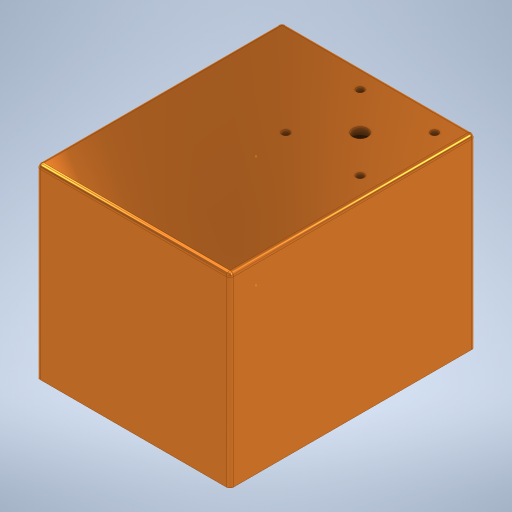
# Autodesk Inventor part: case
Saved by Autodesk Inventor 2023 (Build 270158000, 158)
## iProperties
Created: 2022-11-26
Part Number: case
Material: Gold
Document SubType Name: Modeling
Designer: abdul
Density: 19.3 g/cm^3
Appearance: Metal 1600F Hot
Author: abdul
Autodesk Inventor part; units mm, degrees
ref_plane "YZ Plane" through (0, 0, 0) normal (1, 0, 0) x (0, 1, 0)
ref_plane "XZ Plane" through (0, 0, 0) normal (0, 1, 0) x (-1, 0, 0)
ref_plane "XY Plane" through (0, 0, 0) normal (0, 0, 1) x (1, 0, 0)
sketch "Sketch1" plane through (0, 0, 0) normal (0, 1, 0) x (-1, 0, 0)
  line L0 (130, 165) -> (-130, 165)
  line L1 (-130, 165) -> (-130, -165)
  line L2 (-130, -165) -> (130, -165)
  line L3 (130, -165) -> (130, 165)
  point P0 (0, 0)
  point P1 (0, -165)
  point P2 (-130, 0)
  dimension "d0" = 260
  dimension "d1" = 330
  constraints: 8 end point, 2 midpoint, 2 parallel, 1 horizontal, 1 horizontal alignment, 1 perpendicular, 1 vertical alignment
  measures "d0" distance of L2.end L1.end
  measures "d1" distance of L1.end L0.end
extrude "Extrusion1" add sketch "Sketch1" along normal blind 250
sketch "Sketch2" plane through (0, 0, 0) normal (0, -1, 0) x (1, 0, 0)
  line L0 (-120, 155) -> (120, 155)
  line L1 (120, 155) -> (120, -155)
  line L2 (120, -155) -> (-120, -155)
  line L3 (-120, -155) -> (-120, 155)
  line L4 (-130, 165) -> (130, 165) projected
  line L5 (130, 165) -> (130, -165) projected
  point P0 (0, 0)
  point P1 (0, 155)
  point P2 (-120, 0)
  dimension "d4" = 10
  dimension "d5" = 10
  constraints: 8 end point, 2 midpoint, 2 parallel, 1 horizontal, 1 horizontal alignment, 1 perpendicular, 1 vertical alignment
  measures "d4" distance between parallel lines of L4 L0
  measures "d5" distance between parallel lines of L5 L1
extrude "Extrusion2" cut sketch "Sketch2" against normal blind 240
fillet "Fillet1" radius 5 8 edges at (0, 250, 165) (-130, 250, 0) (130, 250, 0) (0, 250, -165) (130, 125, -165) (130, 125, 165) (-130, 125, 165) (-130, 125, -165)
sketch "Sketch3" plane through (0, 250, 0) normal (0, 1, 0) x (1, 0, 0)
  circle A0 centre (2.5, 37.5) radius 5
  circle A1 centre (2.5, 137.5) radius 5
  circle A2 centre (102.5, 37.5) radius 5
  circle A3 centre (102.5, 137.5) radius 5
  line L0 (125, 160) -> (125, -160) projected
  line L1 (-125, 160) -> (125, 160) projected
  circle A4 centre (52.5, 87.5) radius 10
  point P0 (0, 0)
  dimension "d9" = 10
  dimension "d10" = 10
  dimension "d11" = 10
  dimension "d12" = 10
  dimension "d13" = 100
  dimension "d14" = 100
  dimension "d15" = 22.5
  dimension "d16" = 22.5
  dimension "d19" = 20
  dimension "d20" = 50
  dimension "d21" = 50
  constraints: 5 centre point, 2 horizontal alignment, 2 vertical alignment
  measures "d9" diameter of A0
  measures "d10" diameter of A1
  measures "d11" diameter of A2
  measures "d12" diameter of A3
  measures "d13" distance of A3.centre A2.centre
  measures "d14" distance of A2.centre A0.centre
  measures "d15" distance from line of L0 A2.centre
  measures "d16" distance from line of L1 A3.centre
  measures "d19" diameter of A4
  measures "d20" horizontal distance of A0.centre A4.centre
  measures "d21" horizontal distance of A3.centre A4.centre
extrude "Extrusion3" cut sketch "Sketch3" against normal blind 8
sketch "Sketch4" plane through (52.5, 242, -87.5) normal (0, 1, 0) x (1, 0, 0)
  circle A0 centre (0, 0) radius 10 projected
  circle A1 centre (0, 0) radius 15
  point P0 (-52.5, -87.5)
  constraints: 1 centre point, 1 coincident
extrude "Extrusion4" cut sketch "Sketch4" against normal up to next contours A0
sketch "Sketch5" plane through (0, 240, 0) normal (0, -1, 0) x (1, 0, 0)
  line L0 (87.5, -117.5) -> (17.5, -117.5)
  line L1 (17.5, -117.5) -> (17.5, -57.5)
  line L2 (17.5, -57.5) -> (87.5, -57.5)
  line L3 (87.5, -57.5) -> (87.5, -117.5)
  line L4 (120, -155) -> (-120, -155) projected
  circle A0 centre (52.5, -87.5) radius 15
  circle A1 centre (52.5, -87.5) radius 10 projected
  point P0 (0, 0)
  point P1 (17.5, -87.5)
  point P2 (52.5, -57.5)
  point P3 (52.5, -117.5)
  dimension "d24" = 70
  dimension "d25" = 60
  dimension "d52" = 70
  constraints: 8 end point, 3 midpoint, 2 vertical alignment, 1 centre point, 1 coincident, 1 horizontal alignment, 1 parallel, 1 perpendicular
  measures "d24" distance of L1.end L2.end
  measures "d25" distance of L0.end L1.end
  measures "d52" distance of L0.start L0.end
extrude "Extrusion5" add sketch "Sketch5" along normal blind 150 contours L0 L1 L2 L3
sketch "Sketch7" plane through (0, 90, 0) normal (0, -1, 0) x (1, 0, 0)
  line L0 (85, -105) -> (20, -105)
  line L1 (20, -105) -> (20, -70)
  line L2 (20, -70) -> (85, -70)
  line L3 (85, -70) -> (85, -105)
  line L4 (17.5, -117.5) -> (87.5, -117.5) projected
  line L5 (17.5, -57.5) -> (17.5, -117.5) projected
  point P0 (0, 0)
  point P1 (52.5, -105)
  point P2 (52.5, -117.5)
  point P3 (52.5, -117.5)
  point P4 (17.5, -87.5)
  point P5 (20, -87.5)
  point P6 (100, -102.5)
  dimension "d28" = 65
  dimension "d29" = 35
  constraints: 8 end point, 3 midpoint, 2 parallel, 1 horizontal, 1 horizontal alignment, 1 perpendicular, 1 vertical alignment, 3 other
  measures "d28" distance of L1.end L2.end
  measures "d29" distance of L0.end L1.end
extrude "Extrusion6" cut sketch "Sketch7" against normal blind 150
sketch "Sketch8" plane through (0, 240, 0) normal (0, -1, 0) x (1, 0, 0)
  point P0 (0, 0)
sketch "Sketch9" plane through (0, 240, 0) normal (0, -1, 0) x (1, 0, 0)
  circle A0 centre (67, -87.5) radius 2.5
  circle A1 centre (38, -87.5) radius 2.5
  circle A2 centre (52.5, -87.5) radius 10
  circle A3 centre (52.5, -87.5) radius 10 projected
  point P0 (0, 0)
  dimension "d32" = 5
  dimension "d33" = 5
  dimension "d43" = 14.5
  dimension "d44" = 14.5
  constraints: 3 centre point, 2 horizontal alignment, 1 coincident
  measures "d32" diameter of A0
  measures "d33" diameter of A1
  measures "d43" distance of A0.centre A2.centre
  measures "d44" distance of A2.centre A1.centre
extrude "Extrusion7" add sketch "Sketch9" along normal up to surface (150 mm away) contours A0 | A1
fillet "Fillet2" radius 15 4 edges at (20, 165, -70) (20, 165, -105) (85, 165, -70) (85, 165, -105)
sketch "Sketch10" plane through (0, 90, 0) normal (0, -1, 0) x (1, 0, 0)
  point P0 (0, 0)
sketch "Sketch11" plane through (0, 90, 0) normal (0, -1, 0) x (1, 0, 0)
  line L0 (18.5, -58.5) -> (86.5, -58.5)
  line L1 (86.5, -58.5) -> (86.5, -116.5)
  line L2 (86.5, -116.5) -> (18.5, -116.5)
  line L3 (18.5, -116.5) -> (18.5, -58.5)
  line L4 (17.5, -57.5) -> (17.5, -117.5) projected
  line L5 (87.5, -117.5) -> (87.5, -57.5) projected
  line L6 (87.5, -57.5) -> (17.5, -57.5) projected
  line L7 (17.5, -117.5) -> (87.5, -117.5) projected
  point P0 (0, 0)
  point P1 (100, -42.5)
  point P2 (100, -102.5)
  dimension "d46" = 1
  dimension "d47" = 1
  dimension "d48" = 1
  dimension "d49" = 1
  constraints: 8 end point, 2 parallel, 1 horizontal, 1 perpendicular, 2 other
  measures "d46" distance between parallel lines of L4 L3
  measures "d47" distance between parallel lines of L5 L1
extrude "Extrusion8" add sketch "Sketch11" along normal blind 5
sketch "Sketch12" plane through (-120, 0, 155) normal (1, 0, 0) x (0, 0, -1)
  line L0 (315, 0) -> (165, 0)
  line L1 (165, 0) -> (165, 60)
  line L2 (165, 60) -> (315, 60)
  line L3 (315, 60) -> (315, 0)
  line L4 (315, 245) -> (315, 0) projected
  point P0 (155, 0)
  dimension "d53" = 150
  dimension "d54" = 60
  dimension "d57" = 0
  constraints: 8 end point, 2 parallel, 1 horizontal, 1 perpendicular
  measures "d53" distance of L1.end L2.end
  measures "d54" distance of L0.end L1.end
  measures "d57" distance between parallel lines of L4 L3
extrude "Extrusion9" add sketch "Sketch12" along normal blind 130
sketch "Sketch15" plane through (0, 85, 0) normal (0, -1, 0) x (1, 0, 0)
  line L0 (97.9773, -47.1324) -> (13.5699, -47.1324)
  line L1 (13.5699, -47.1324) -> (13.5699, -120.1648)
  line L2 (13.5699, -120.1648) -> (97.9773, -120.1648)
  line L3 (97.9773, -120.1648) -> (97.9773, -47.1324)
  point P0 (0, 0)
  constraints: 8 end point, 2 parallel, 1 horizontal, 1 perpendicular
extrude "Extrusion11" cut sketch "Sketch15" against normal blind 50
sketch "Sketch17" plane through (0, 135, 0) normal (0, -1, 0) x (1, 0, 0)
  line L0 (87.5, -57.5) -> (87.5, -117.5) projected
  line L1 (87.5, -117.5) -> (17.5, -117.5) projected
  line L2 (87.5, -57.5) -> (17.5, -57.5)
  line L3 (17.5, -57.5) -> (17.5, -117.5)
  line L4 (17.5, -117.5) -> (87.5, -117.5)
  line L5 (87.5, -117.5) -> (87.5, -57.5)
  line L6 (87, -58) -> (18, -58)
  line L7 (18, -58) -> (18, -117)
  line L8 (18, -117) -> (87, -117)
  line L9 (87, -117) -> (87, -58)
  point P0 (0, 0)
  dimension "d70" = 0.5
  dimension "d71" = 0.5
  dimension "d72" = 0.5
  dimension "d73" = 0.5
  constraints: 16 end point, 4 parallel, 2 horizontal, 2 perpendicular
  measures "d70" distance between parallel lines of L0 L9
  measures "d71" distance between parallel lines of L2 L6
  measures "d72" distance between parallel lines of L1 L8
  measures "d73" distance between parallel lines of L3 L7
extrude "Extrusion12" cut sketch "Sketch17" against normal blind 5 contours L9 L8 L7 L6
chamfer "Chamfer2" distance 0.2 angle 45 4 edges at (52.5, 135, -117) (87, 135, -87.5) (52.5, 135, -58) (18, 135, -87.5)
sketch "Sketch18" plane through (-120, 240, -155) normal (0, 0, 1) x (1, 0, 0)
  line L0 (-10.236, -242) -> (249.4607, -242) projected
  line L1 (230, -242) -> (130, -242)
  line L2 (130, -242) -> (130, -212)
  line L3 (130, -212) -> (230, -212)
  line L4 (230, -212) -> (230, -242)
  line L5 (250, 5) -> (250, -240) projected
  line L6 (245, -240) -> (245, 5) projected
  point P0 (120, -240)
  dimension "d79" = 100
  dimension "d80" = 30
  dimension "d91" = 15
  constraints: 8 end point, 2 parallel, 1 horizontal, 1 perpendicular, 1 point on line
  measures "d79" distance of L2.end L3.end
  measures "d80" distance of L1.end L2.end
  measures "d91" distance between parallel lines of L6 L4
extrude "Extrusion13" add sketch "Sketch18" along normal blind 150
sketch "Sketch19" plane through (125, 245, -165) normal (0, 0, -1) x (-1, 0, 0)
  line L0 (115, -247) -> (15, -247) projected
  line L1 (115, -217) -> (115, -247) projected
  line L2 (115, -247) -> (15, -247) projected
  line L3 (15, -247) -> (15, -217) projected
  line L4 (15, -217) -> (115, -217) projected
  line L5 (20, -222) -> (110, -222)
  line L6 (110, -222) -> (110, -265.9747)
  line L7 (110, -265.9747) -> (20, -265.9747)
  line L8 (20, -265.9747) -> (20, -222)
  point P0 (125, -245)
  dimension "d84" = 5
  dimension "d85" = 5
  dimension "d87" = 5
  constraints: 8 end point, 2 parallel, 1 horizontal, 1 perpendicular
  measures "d84" distance between parallel lines of L4 L5
  measures "d85" distance between parallel lines of L3 L8
  measures "d87" distance between parallel lines of L6 L1
extrude "Extrusion14" cut sketch "Sketch19" against normal blind 140 contours L6 L7 L8 L0 | L0 L8 L5 L6
fillet "Fillet3" radius 5 3 edges at (105, 11.5, -165) (60, 23, -165) (15, 11.5, -165)
body "Solid1"
